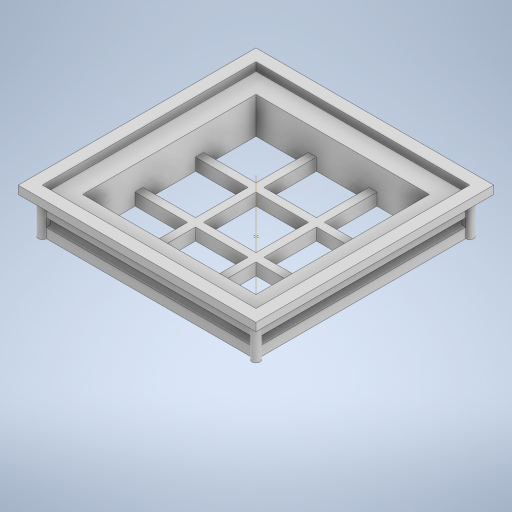
# Autodesk Inventor part: sensor_soldering_mold
Saved by Autodesk Inventor 2023.1 (Build 271208000, 208)
## iProperties
Created: 2022-08-08
Part Number: sensor_soldering_mold
Material: Generic
Document SubType Name: Modeling
Designer: fraaw
Density: 1 g/cm^3
Appearance: Default
Author: fraaw
## iProperties of the stored document sensor_soldering_mold_3DPrint.ipt
Created: 2022-08-08
Part Number: sensor_soldering_mold_3DPrint
Material: Generic
Document SubType Name: Modeling
Designer: fraaw
Density: 1 g/cm^3
Appearance: Default
Author: fraaw
Autodesk Inventor part; units mm, degrees
ref_plane "YZ Plane" through (0, 0, 0) normal (1, 0, 0) x (0, 1, 0)
ref_plane "XZ Plane" through (0, 0, 0) normal (0, 1, 0) x (-1, 0, 0)
ref_plane "XY Plane" through (0, 0, 0) normal (0, 0, 1) x (1, 0, 0)
sketch "Sketch1" plane through (0, 0, 0) normal (0, 1, 0) x (-1, 0, 0)
  line L0 (3.25, 3.25) -> (-3.25, 3.25)
  line L1 (-3.25, 3.25) -> (-3.25, -3.25)
  line L2 (-3.25, -3.25) -> (3.25, -3.25)
  line L3 (3.25, -3.25) -> (3.25, 3.25)
  line L4 (3.25, 3.25) -> (-3.25, -3.25) construction
  line L5 (-3.25, 3.25) -> (3.25, -3.25) construction
  line L6 (3.25, 10.75) -> (-3.25, 10.75)
  line L7 (-3.25, 10.75) -> (-3.25, 4.25)
  line L8 (-3.25, 4.25) -> (3.25, 4.25)
  line L9 (3.25, 4.25) -> (3.25, 10.75)
  line L10 (3.25, 10.75) -> (-3.25, 4.25) construction
  line L11 (-3.25, 10.75) -> (3.25, 4.25) construction
  line L12 (3.25, -4.25) -> (-3.25, -4.25)
  line L13 (-3.25, -4.25) -> (-3.25, -10.75)
  line L14 (-3.25, -10.75) -> (3.25, -10.75)
  line L15 (3.25, -10.75) -> (3.25, -4.25)
  line L16 (3.25, -4.25) -> (-3.25, -10.75) construction
  line L17 (-3.25, -4.25) -> (3.25, -10.75) construction
  line L18 (3.25, 3.25) -> (-3.25, 3.25)
  line L19 (-3.25, 3.25) -> (-3.25, -3.25)
  line L20 (-3.25, -3.25) -> (3.25, -3.25)
  line L21 (3.25, -3.25) -> (3.25, 3.25)
  line L22 (3.25, 3.25) -> (-3.25, -3.25) construction
  line L23 (-3.25, 3.25) -> (3.25, -3.25) construction
  line L24 (10.75, -3.25) -> (10.75, 3.25)
  line L25 (10.75, -3.25) -> (10.75, 3.25)
  line L26 (10.75, 3.25) -> (4.25, -3.25) construction
  line L27 (10.75, 3.25) -> (4.25, -3.25) construction
  line L28 (4.25, -3.25) -> (10.75, -3.25)
  line L29 (4.25, 3.25) -> (10.75, -3.25) construction
  line L30 (4.25, 3.25) -> (10.75, -3.25) construction
  line L31 (4.25, 3.25) -> (4.25, -3.25)
  line L32 (4.25, 3.25) -> (4.25, -3.25)
  line L33 (10.75, 3.25) -> (4.25, 3.25)
  line L34 (10.75, 3.25) -> (4.25, 3.25)
  line L35 (4.25, 4.25) -> (10.75, 4.25)
  line L36 (10.75, 4.25) -> (10.75, 10.75)
  line L37 (10.75, 10.75) -> (4.25, 4.25) construction
  line L38 (4.25, 10.75) -> (10.75, 4.25) construction
  line L39 (4.25, 10.75) -> (4.25, 4.25)
  line L40 (10.75, 10.75) -> (4.25, 10.75)
  line L41 (4.25, -3.25) -> (10.75, -3.25)
  line L42 (10.75, -4.25) -> (4.25, -4.25)
  line L43 (4.25, -4.25) -> (4.25, -10.75)
  line L44 (10.75, -4.25) -> (4.25, -10.75) construction
  line L45 (4.25, -10.75) -> (10.75, -10.75)
  line L46 (4.25, -4.25) -> (10.75, -10.75) construction
  line L47 (10.75, -10.75) -> (10.75, -4.25)
  line L48 (-4.25, -3.25) -> (-4.25, 3.25)
  line L49 (-4.25, -3.25) -> (-4.25, 3.25)
  line L50 (-4.25, 3.25) -> (-10.75, -3.25) construction
  line L51 (-4.25, 3.25) -> (-10.75, -3.25) construction
  line L52 (-10.75, -3.25) -> (-4.25, -3.25)
  line L53 (-10.75, 3.25) -> (-4.25, -3.25) construction
  line L54 (-10.75, 3.25) -> (-4.25, -3.25) construction
  line L55 (-10.75, 3.25) -> (-10.75, -3.25)
  line L56 (-10.75, 3.25) -> (-10.75, -3.25)
  line L57 (-4.25, 3.25) -> (-10.75, 3.25)
  line L58 (-4.25, 3.25) -> (-10.75, 3.25)
  line L59 (-10.75, 4.25) -> (-4.25, 4.25)
  line L60 (-4.25, 4.25) -> (-4.25, 10.75)
  line L61 (-4.25, 10.75) -> (-10.75, 4.25) construction
  line L62 (-10.75, 10.75) -> (-4.25, 4.25) construction
  line L63 (-10.75, 10.75) -> (-10.75, 4.25)
  line L64 (-4.25, 10.75) -> (-10.75, 10.75)
  line L65 (-10.75, -3.25) -> (-4.25, -3.25)
  line L66 (-4.25, -4.25) -> (-10.75, -4.25)
  line L67 (-10.75, -4.25) -> (-10.75, -10.75)
  line L68 (-4.25, -4.25) -> (-10.75, -10.75) construction
  line L69 (-10.75, -10.75) -> (-4.25, -10.75)
  line L70 (-10.75, -4.25) -> (-4.25, -10.75) construction
  line L71 (-4.25, -10.75) -> (-4.25, -4.25)
  line L72 (3.25, -3.25) -> (3.25, 3.25)
  line L73 (3.25, -3.25) -> (3.25, 3.25)
  line L74 (3.25, 3.25) -> (-3.25, -3.25) construction
  line L75 (3.25, 3.25) -> (-3.25, -3.25) construction
  line L76 (-3.25, -3.25) -> (3.25, -3.25)
  line L77 (-3.25, 3.25) -> (3.25, -3.25) construction
  line L78 (-3.25, 3.25) -> (3.25, -3.25) construction
  line L79 (-3.25, 3.25) -> (-3.25, -3.25)
  line L80 (-3.25, 3.25) -> (-3.25, -3.25)
  line L81 (3.25, 3.25) -> (-3.25, 3.25)
  line L82 (3.25, 3.25) -> (-3.25, 3.25)
  line L83 (-3.25, 4.25) -> (3.25, 4.25)
  line L84 (3.25, 4.25) -> (3.25, 10.75)
  line L85 (3.25, 10.75) -> (-3.25, 4.25) construction
  line L86 (-3.25, 10.75) -> (3.25, 4.25) construction
  line L87 (-3.25, 10.75) -> (-3.25, 4.25)
  line L88 (3.25, 10.75) -> (-3.25, 10.75)
  line L89 (-3.25, -3.25) -> (3.25, -3.25)
  line L90 (3.25, -4.25) -> (-3.25, -4.25)
  line L91 (-3.25, -4.25) -> (-3.25, -10.75)
  line L92 (3.25, -4.25) -> (-3.25, -10.75) construction
  line L93 (-3.25, -10.75) -> (3.25, -10.75)
  line L94 (-3.25, -4.25) -> (3.25, -10.75) construction
  line L95 (3.25, -10.75) -> (3.25, -4.25)
  line L96 (13.25, 13.25) -> (-13.25, 13.25)
  line L97 (-13.25, 13.25) -> (-13.25, -13.25)
  line L98 (-13.25, -13.25) -> (13.25, -13.25)
  line L99 (13.25, -13.25) -> (13.25, 13.25)
  line L100 (13.25, 13.25) -> (-13.25, -13.25) construction
  line L101 (-13.25, 13.25) -> (13.25, -13.25) construction
  point P0 (0, 0)
  point P1 (0, 7.5)
  point P2 (0, -7.5)
  point P3 (0, 0)
  point P4 (7.5, 0)
  point P5 (7.5, 0)
  point P6 (7.5, 7.5)
  point P7 (7.5, -7.5)
  point P8 (-7.5, 0)
  point P9 (-7.5, 0)
  point P10 (-7.5, 7.5)
  point P11 (-7.5, -7.5)
  point P12 (0, 0)
  point P13 (0, 0)
  point P14 (0, 7.5)
  point P15 (0, -7.5)
  dimension "d0" = 6.5
  dimension "d1" = 6.5
  dimension "d4" = 7.5
  dimension "d7" = 7.5
  dimension "d12" = 7.5
  dimension "d15" = 7.5
  dimension "d18" = 2.5
  constraints: 204 end point, 4 collinear, 4 horizontal, 4 midpoint, 4 parallel, 2 perpendicular, 2 vertical, 1 point on line, 161 other
  measures "d0" distance of L1.end L2.end
  measures "d1" distance of L2.end L0.start
  measures "d4" distance of L0.start L6.start
  measures "d7" distance of L0.start L12.start
  measures "d12" distance of point (0, 0) point (7.5, 0)
  measures "d15" distance of point (0, 0) point (-7.5, 0)
  measures "d18" distance between parallel lines of L45 L98
extrude "Extrusion1" add sketch "Sketch1" along normal blind 1.5
sketch "Sketch4" plane through (0, 1.5, 0) normal (0, 1, 0) x (1, 0, 0)
  line L0 (13.25, 13.25) -> (-13.25, 13.25) projected
  line L1 (-13.25, 13.25) -> (-13.25, -13.25) projected
  line L2 (13.25, -13.25) -> (13.25, 13.25) projected
  line L3 (-13.25, -13.25) -> (13.25, -13.25) projected
  line L4 (-10.75, 10.75) -> (10.75, 10.75)
  line L5 (10.75, 10.75) -> (10.75, -10.75)
  line L6 (10.75, -10.75) -> (-10.75, -10.75)
  line L7 (-10.75, -10.75) -> (-10.75, 10.75)
  point P0 (0, 0)
  dimension "d31" = 2.5
  constraints: 8 end point, 3 other
  measures "d31" distance between parallel lines of L7 L1
extrude "Extrusion3" add sketch "Sketch4" along normal blind 3
sketch "Sketch5" plane through (0, 4.5, 0) normal (0, 1, 0) x (1, 0, 0)
  line L0 (-13.25, 13.25) -> (-13.25, -13.25) projected
  line L1 (-13.25, -13.25) -> (13.25, -13.25) projected
  line L2 (13.25, -13.25) -> (13.25, 13.25) projected
  line L3 (13.25, 13.25) -> (-13.25, 13.25) projected
  line L4 (-10.75, 10.75) -> (10.75, 10.75) projected
  line L5 (10.75, 10.75) -> (10.75, -10.75) projected
  line L6 (10.75, -10.75) -> (-10.75, -10.75) projected
  line L7 (-10.75, -10.75) -> (-10.75, 10.75) projected
  line L8 (-14.75, 14.75) -> (-14.75, -14.75)
  line L9 (-14.75, -14.75) -> (14.75, -14.75)
  line L10 (14.75, -14.75) -> (14.75, 14.75)
  line L11 (14.75, 14.75) -> (-14.75, 14.75)
  point P0 (0, 0)
  dimension "d34" = 1.5
  constraints: 8 end point, 3 other
  measures "d34" distance between parallel lines of L3 L11
extrude "Extrusion4" add sketch "Sketch5" along normal blind 1 contours L11 L10 L9 L8
sketch "Sketch7" plane through (0, 0, 0) normal (0, -1, 0) x (1, 0, 0)
  line L0 (-13.25, 13.25) -> (-13.25, -13.25) projected
  circle A0 centre (-13.25, 13.25) radius 0.5
  circle A1 centre (-13.25, -13.25) radius 0.5
  line L1 (13.25, 13.25) -> (13.25, -13.25) projected
  circle A2 centre (13.25, -13.25) radius 0.5
  circle A3 centre (13.25, 13.25) radius 0.5
  point P0 (0, 0)
  dimension "d37" = 1
  dimension "d38" = 1
  dimension "d39" = 1
  dimension "d40" = 1
  constraints: 4 centre point, 2 coincident
  measures "d37" diameter of A0
  measures "d38" diameter of A1
  measures "d39" diameter of A3
  measures "d40" diameter of A2
extrude "Extrusion5" add sketch "Sketch7" against normal up to surface (4.5 mm away)
sketch "Sketch10" plane through (-12.75, 0, 13.25) normal (0, 0, 1) x (1, 0, 0)
  line L0 (0, 0) -> (0, 4.5) projected
  line L1 (25.5, 4.5) -> (25.5, 0) projected
  line L2 (0, 2.25) -> (25.5, 2.25)
  line L3 (25.5, 2.25) -> (25.5, 1.25)
  line L4 (25.5, 1.25) -> (0, 1.25)
  line L5 (0, 1.25) -> (0, 2.25)
  point P0 (12.75, 0)
  point P1 (0, 1.25)
  dimension "d43" = 1
  constraints: 8 end point, 2 parallel, 1 horizontal, 1 midpoint, 1 perpendicular, 1 point on line
  measures "d43" distance between parallel lines of L4 L2
extrude "Extrusion6" cut sketch "Sketch10" against normal blind 1
sketch "Sketch11" plane through (0, 0, 0) normal (0, -1, 0) x (1, 0, 0)
  point P0 (0, 0)
  point P1 (0, 0)
  constraints: 1 coincident
pattern_circular "Circular Pattern1" count 4 over 360 about axis through (0, 0, 0) along (0, -1, 0) of "Extrusion6"
equation "\"d1\" = d0"
body "Solid1"
